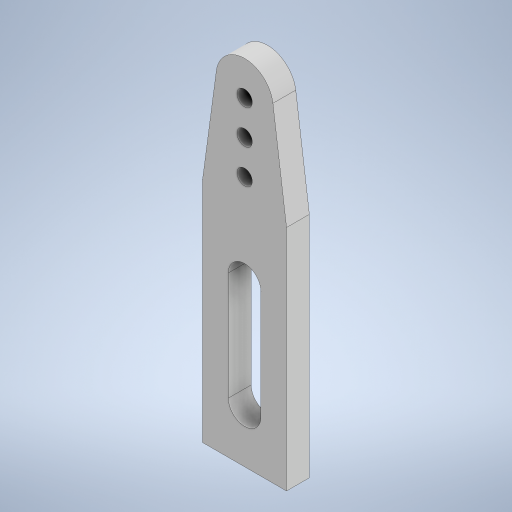
# Autodesk Inventor part: Standard Servo Horn - Linear Arm
Saved by Autodesk Inventor 2023 (Build 270158000, 158)
## iProperties
Created: 2023-09-01
Part Number: Standard Servo Horn - Linear Arm
Material: Generic
Document SubType Name: Modeling
Designer: Nate
Density: 1 g/cm^3
Appearance: Default
Author: Nate
Autodesk Inventor part; units mm, degrees
ref_plane "YZ Plane" through (0, 0, 0) normal (1, 0, 0) x (0, 1, 0)
ref_plane "XZ Plane" through (0, 0, 0) normal (0, 1, 0) x (-1, 0, 0)
ref_plane "XY Plane" through (0, 0, 0) normal (0, 0, 1) x (1, 0, 0)
sketch "Sketch1" plane through (0, 0, 0) normal (0, 0, 1) x (1, 0, 0)
  line L0 (0, 0) -> (7.35, 0)
  line L1 (7.35, 0) -> (7.35, 20)
  line L2 (7.35, 20) -> (0, 20)
  line L3 (0, 20) -> (0, 0)
  circle A0 centre (3.68, 28.5) radius 2.5
  line L4 (1.2028, 28.8372) -> (0, 20)
  line L5 (6.1575, 28.8344) -> (7.35, 20)
  circle A1 centre (3.68, 28) radius 0.67
  circle A2 centre (3.68, 4.5) radius 1.43
  circle A3 centre (3.68, 14) radius 1.43
  circle A4 centre (3.68, 25) radius 0.67
  circle A5 centre (3.68, 22) radius 0.67
  line L6 (2.25, 4.5) -> (2.25, 14)
  line L7 (5.11, 14) -> (5.11, 4.5)
  point P0 (5.11, 4.5)
  dimension "d0" = 7.35
  dimension "d1" = 20
  dimension "d2" = 5
  dimension "d3" = 28.5
  dimension "d4" = 3.68
  dimension "d5" = 1.34
  dimension "d6" = 2.86
  dimension "d7" = 2.86
  dimension "d8" = 1.34
  dimension "d9" = 1.34
  dimension "d10" = 28
  dimension "d11" = 3.68
  dimension "d12" = 25
  dimension "d13" = 3.68
  dimension "d14" = 3.68
  dimension "d15" = 22
  dimension "d16" = 14
  dimension "d17" = 4.5
  dimension "d18" = 3.68
  dimension "d19" = 3.68
  constraints: 16 end point, 8 point on circle, 6 centre point, 3 parallel, 3 tangent, 1 horizontal, 1 perpendicular, 1 vertical
  measures "d0" distance of L2.end L1.end
  measures "d1" distance of L1.end L0.end
  measures "d2" diameter of A0
  measures "d3" distance from line of A0.centre L0
  measures "d4" horizontal distance of L0.start A0.centre
  measures "d5" diameter of A1
  measures "d6" diameter of A2
  measures "d7" diameter of A3
  measures "d8" diameter of A4
  measures "d9" diameter of A5
  measures "d10" distance from line of L0 A1.centre
  measures "d11" distance from line of L3 A1.centre
  measures "d12" distance from line of L0 A4.centre
  measures "d13" distance from line of L3 A4.centre
  measures "d14" distance from line of L3 A5.centre
  measures "d15" distance from line of L0 A5.centre
  measures "d16" distance from line of L0 A3.centre
  measures "d17" distance from line of L0 A2.centre
  measures "d18" distance from line of L3 A2.centre
  measures "d19" distance from line of L3 A3.centre
extrude "Extrusion1" add sketch "Sketch1" along normal blind 2
body "Solid1"
